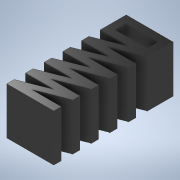
# Autodesk Inventor part: resorte
Saved by Autodesk Inventor 2021.5 (Build 255421000, 421)
## iProperties
Created: 2024-11-28
Part Number: resorte
Material: Genérico
Document SubType Name: Modeling
Designer: Joho_
Density: 1 g/cm^3
Appearance: Valor por defecto
Author: Joho_
Autodesk Inventor part; units mm, degrees
ref_plane "YZ Plane" through (0, 0, 0) normal (1, 0, 0) x (0, 1, 0)
ref_plane "XZ Plane" through (0, 0, 0) normal (0, 1, 0) x (-1, 0, 0)
ref_plane "XY Plane" through (0, 0, 0) normal (0, 0, 1) x (1, 0, 0)
sketch "Boceto1" plane through (0, 0, 0) normal (0, 0, 1) x (1, 0, 0)
  circle A0 centre (0, 0) radius 8.9
  line L0 (6.2933, -6.2933) -> (-6.2933, -6.2933)
  line L1 (-6.2933, -6.2933) -> (-6.2933, 6.2933)
  line L2 (-6.2933, 6.2933) -> (6.2933, 6.2933)
  line L3 (6.2933, 6.2933) -> (6.2933, -6.2933)
  dimension "d0" = 17.8
  dimension "d1" = 12.5865
  dimension "d2" = 12.5865
  constraints: 8 end point, 2 parallel, 1 centre point, 1 coincident, 1 horizontal, 1 perpendicular
  measures "d0" diameter of A0
  measures "d1" distance of L1.end L2.end
  measures "d2" distance of L0.end L1.end
extrude "Extrusión1" add sketch "Boceto1" along normal blind 32 contours L3 L0 L1 L2
sketch "Boceto2" plane through (0, 0, 0) normal (0, 1, 0) x (-1, 0, 0)
  line L0 (6.2933, 0) -> (-6.2933, 0)
  line L1 (-6.2933, 0) -> (-6.2933, 2)
  line L2 (-6.2933, 2) -> (6.2933, 2)
  line L3 (6.2933, 2) -> (6.2933, 0)
  line L4 (6.2933, 5) -> (-6.2933, 5)
  line L5 (-6.2933, 5) -> (-6.2933, 7)
  line L6 (-6.2933, 7) -> (6.2933, 7)
  line L7 (6.2933, 7) -> (6.2933, 5)
  line L8 (6.2933, 10) -> (-6.2933, 10)
  line L9 (-6.2933, 10) -> (-6.2933, 12)
  line L10 (-6.2933, 12) -> (6.2933, 12)
  line L11 (6.2933, 12) -> (6.2933, 10)
  line L12 (6.2933, 15) -> (-6.2933, 15)
  line L13 (-6.2933, 15) -> (-6.2933, 17)
  line L14 (-6.2933, 17) -> (6.2933, 17)
  line L15 (6.2933, 17) -> (6.2933, 15)
  line L16 (6.2933, 20) -> (-6.2933, 20)
  line L17 (-6.2933, 20) -> (-6.2933, 22)
  line L18 (-6.2933, 22) -> (6.2933, 22)
  line L19 (6.2933, 22) -> (6.2933, 20)
  line L20 (6.2933, 25) -> (-6.2933, 25)
  line L21 (-6.2933, 25) -> (-6.2933, 27)
  line L22 (-6.2933, 27) -> (6.2933, 27)
  line L23 (6.2933, 27) -> (6.2933, 25)
  line L24 (6.2933, 30) -> (-6.2933, 30)
  line L25 (-6.2933, 30) -> (-6.2933, 32)
  line L26 (-6.2933, 32) -> (6.2933, 32)
  line L27 (6.2933, 32) -> (6.2933, 30)
  line L28 (-6.2933, 0) -> (6.2933, 0) projected
  line L29 (-6.2933, 0) -> (6.2933, 5)
  line L30 (-6.2933, 1.883) -> (6.2933, 6.883)
  line L31 (-6.2933, 6.883) -> (6.2933, 11.883)
  line L32 (-6.2933, 5) -> (6.2933, 10)
  line L33 (-6.2933, 11.883) -> (6.2933, 16.883)
  line L34 (-6.2933, 10) -> (6.2933, 15)
  line L35 (-6.2933, 16.883) -> (6.2933, 21.883)
  line L36 (-6.2933, 15) -> (6.2933, 20)
  line L37 (-6.2933, 21.883) -> (6.2933, 26.883)
  line L38 (-6.2933, 20) -> (6.2933, 25)
  line L39 (-6.2933, 26.883) -> (6.2933, 31.883)
  line L40 (-6.2933, 25) -> (6.2933, 30)
  line L41 (6.2933, 0) -> (4.2933, 0)
  line L42 (4.2933, 0) -> (4.2933, 7)
  line L43 (4.2933, 7) -> (6.2933, 7)
  line L44 (6.2933, 7) -> (6.2933, 0)
  line L45 (-6.2933, 0) -> (-4.2933, 0)
  line L46 (-4.2933, 0) -> (-4.2933, 7)
  line L47 (-4.2933, 7) -> (-6.2933, 7)
  line L48 (-6.2933, 7) -> (-6.2933, 0)
  point P0 (0, 0)
  point P1 (0, 5)
  point P2 (0, 10)
  point P3 (0, 15)
  point P4 (0, 20)
  point P5 (0, 25)
  point P6 (0, 30)
  point P7 (1.5531, 30)
  point P8 (-5.9988, 27)
  point P9 (1.5531, 25)
  point P10 (-5.9988, 22)
  point P11 (1.5531, 20)
  point P12 (-5.9988, 17)
  point P13 (1.5531, 15)
  point P14 (-5.9988, 12)
  point P15 (1.5531, 10)
  point P16 (-5.9988, 7)
  point P17 (1.5531, 5)
  point P18 (-5.9988, 2)
  point P19 (-1.2586, 2)
  point P20 (-1.2587, 7)
  point P21 (-1.2587, 12)
  point P22 (-1.2587, 17)
  point P23 (-1.2586, 22)
  point P24 (-1.2586, 27)
  point P25 (4.2933, 5)
  point P26 (4.2933, 2)
  point P27 (-4.2933, 2)
  point P28 (-4.2933, 5)
  dimension "d5" = 2
  dimension "d8" = 5
  dimension "d13" = 1.75
  dimension "d16" = 5
  dimension "d23" = 2
  dimension "d24" = 2
  constraints: 96 end point, 5 parallel, 4 point on line, 2 horizontal, 2 perpendicular, 2 vertical, 1 coincident, 1 collinear, 83 other
  measures "d5" distance of L0.end L1.end
  measures "d8" distance of point (0, 0) point (0, 5)
  measures "d13" distance between parallel lines of L29 L30
  measures "d16" distance of L30.start L31.start
  measures "d23" distance of L42.end L43.end
  measures "d24" distance of L47.end L46.end
extrude "Extrusión2" cut sketch "Boceto2" against normal mid plane 30 contours L0 L42 L2 L3 | L0 L46 L29 L2 L42 | L2 L42 L29 L44 | L0 L29 L46 | L29 L42 L4 | L4 L42 L30 L7 | L1 L30 L2 L46 L29 | L46 L2 L29 | L4 L30 L42 | L30 L42 L6 L7 | L1 L2 L30 | L2 L30 L46 | L4 L46 L32 L6 L42 L30 | L48 L4 L46 L30 L2 | L4 L32 L46 | L5 L31 L6 L46 L32 | L46 L6 L32 | L6 L31 L8 L32 | L5 L6 L31 | L8 L31 L11 | L8 L34 L10 L11 L31 | L9 L33 L10 L34 | L9 L10 L33 | L10 L33 L12 L34 | L12 L33 L15 | L12 L36 L14 L15 L33 | L13 L35 L14 L36 | L13 L14 L35 | L14 L35 L16 L36 | L16 L35 L19 | L16 L38 L18 L19 L35 | L17 L37 L18 L38 | L17 L18 L37 | L18 L37 L20 L38 | L20 L37 L23 | L20 L40 L22 L23 L37 | L21 L39 L22 L40 | L21 L22 L39 | L22 L39 L24 L40 | L24 L39 L27 | L24 L25 L26 L27 L39 keep common part
sketch "Boceto3" plane through (0, 0, 0) normal (0, 0, -1) x (-1, 0, 0)
  circle A0 centre (0, 0) radius 2
  dimension "d25" = 4
  constraints: 1 centre point, 1 coincident
  measures "d25" diameter of A0
extrude "Extrusión3" cut sketch "Boceto3" against normal blind 20
